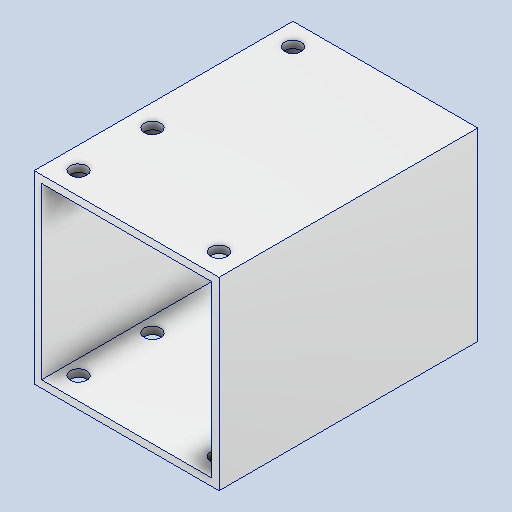
# Autodesk Inventor part: hip
Saved by Autodesk Inventor 2022 (Build 260153000, 153)
## iProperties
Created: 2022-10-09
Part Number: hip
Material: アルミニウム 6061
Document SubType Name: Modeling
Designer: haya
Density: 2.7 g/cm^3
Appearance: アルミニウム - フラット
Mass: 71.8889 g
Surface Area: 276.197 cm^2
Volume: 26.6255 cm^3
Author: haya
Autodesk Inventor part; units mm, degrees
ref_plane "YZ Plane" through (0, 0, 0) normal (1, 0, 0) x (0, 1, 0)
ref_plane "XZ Plane" through (0, 0, 0) normal (0, 1, 0) x (-1, 0, 0)
ref_plane "XY Plane" through (0, 0, 0) normal (0, 0, 1) x (1, 0, 0)
sketch "スケッチ1" plane through (0, 0, 0) normal (0, 0, 1) x (1, 0, 0)
  line L0 (0, 0) -> (50, 0)
  line L1 (50, 0) -> (50, 50)
  line L2 (50, 50) -> (0, 50)
  line L3 (0, 50) -> (0, 0)
  line L4 (2, 48) -> (48, 48)
  line L5 (48, 48) -> (48, 2)
  line L6 (48, 2) -> (2, 2)
  line L7 (2, 2) -> (2, 48)
  dimension "d0" = 50
  dimension "d1" = 50
  dimension "d2" = 2
  constraints: 16 end point, 4 parallel, 2 perpendicular, 1 horizontal, 3 other
  measures "d0" distance of L2.end L0.start
  measures "d1" distance of L0.start L0.end
  measures "d2" distance between parallel lines of L0 L6
extrude "押し出し1" add sketch "スケッチ1" along normal blind 70
sketch "スケッチ2" plane through (0, 50, 0) normal (0, 1, 0) x (1, 0, 0)
  line L0 (50, 0) -> (0, 0) projected
  line L1 (0, 0) -> (0, -70) projected
  line L2 (50, -70) -> (0, -70) projected
  line L3 (50, 0) -> (50, -70) projected
  line L4 (50, -64) -> (0, -64) construction
  point P0 (0, 0)
  point P1 (44, -64)
  point P2 (6, -64)
  dimension "d6" = 6
  dimension "d7" = 38
  dimension "d24" = 6
  constraints: 4 point on line, 2 end point, 1 perpendicular
  measures "d6" distance from line of point (44, -64) L3
  measures "d7" distance of point (6, -64) point (44, -64)
  measures "d24" distance between parallel lines of L4 L2
hole "穴1" at (44, 50, 64) at (6, 50, 64) direction (0, -1, 0) diameter 4.5 end through all
sketch "スケッチ4" plane through (0, 50, 0) normal (0, 1, 0) x (1, 0, 0)
  circle A0 centre (44, -64) radius 2.25 projected
  circle A1 centre (6, -64) radius 2.25 projected
  line L0 (50, 0) -> (0, 0) projected
  line L1 (0, 0) -> (0, -70) projected
  line L2 (50, -70) -> (0, -70) projected
  line L3 (50, 0) -> (50, -70) projected
  line L4 (6, -70) -> (6, 0) construction
  point P0 (0, 0)
  point P1 (6, -6)
  point P2 (6, -44)
  dimension "d25" = 6
  dimension "d26" = 6
  dimension "d27" = 38
  constraints: 4 point on line, 2 end point, 1 perpendicular
  measures "d25" distance between parallel lines of L4 L1
  measures "d26" distance from line of point (6, -6) L0
  measures "d27" distance of point (6, -44) point (6, -6)
hole "穴3" at (6, 50, 6) at (6, 50, 44) direction (0, -1, 0) diameter 4.5 end through all
